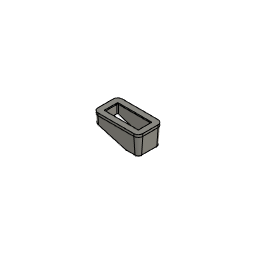
Power Switch Protector (Autodesk Fusion 360 design; units mm, degrees)
Autodesk Fusion 360 part; units mm, degrees
note: some values were not read from the file. Chosen so that the rebuilt part matches the saved one: a direction.
sketch "Sketch1" plane through (0, 0, 0) normal (0, 0, 1) x (-1, 0, 0)
  arc A0 (15.021, -6.6477) -> (15.275, -6.3937) centre (15.021, -6.3937) ccw
  line L0 (15.275, -6.3937) -> (15.275, 6.3937)
  arc A1 (15.275, 6.3937) -> (15.021, 6.6477) centre (15.021, 6.3937) ccw
  line L1 (15.021, 6.6477) -> (-15.021, 6.6477)
  arc A2 (-15.021, 6.6477) -> (-15.275, 6.3937) centre (-15.021, 6.3937) ccw
  line L2 (-15.275, 6.3937) -> (-15.275, -6.3937)
  arc A3 (-15.275, -6.3937) -> (-15.021, -6.6477) centre (-15.021, -6.3937) ccw
  line L3 (-15.021, -6.6477) -> (15.021, -6.6477)
  line L4 (17.675, -6.3937) -> (17.675, 6.3937)
  arc A4 (17.675, 6.3937) -> (15.021, 9.0477) centre (15.021, 6.3937) ccw
  line L5 (15.021, 9.0477) -> (-15.021, 9.0477)
  arc A5 (-15.021, 9.0477) -> (-17.675, 6.3937) centre (-15.021, 6.3937) ccw
  line L6 (-17.675, 6.3937) -> (-17.675, -6.3937)
  arc A6 (-17.675, -6.3937) -> (-15.021, -9.0477) centre (-15.021, -6.3937) ccw
  line L7 (-15.021, -9.0477) -> (15.021, -9.0477)
  arc A7 (15.021, -9.0477) -> (17.675, -6.3937) centre (15.021, -6.3937) ccw
  line L8 (15.675, -6.3937) -> (15.675, 6.3937)
  arc A8 (15.675, 6.3937) -> (15.021, 7.0477) centre (15.021, 6.3937) ccw
  line L9 (15.021, 7.0477) -> (-15.021, 7.0477)
  arc A9 (-15.021, 7.0477) -> (-15.675, 6.3937) centre (-15.021, 6.3937) ccw
  line L10 (-15.675, 6.3937) -> (-15.675, -6.3937)
  arc A10 (-15.675, -6.3937) -> (-15.021, -7.0477) centre (-15.021, -6.3937) ccw
  line L11 (-15.021, -7.0477) -> (15.021, -7.0477)
  arc A11 (15.021, -7.0477) -> (15.675, -6.3937) centre (15.021, -6.3937) ccw
  line L12 (15.021, 10.1477) -> (-15.021, 10.1477)
  arc A12 (-15.021, 10.1477) -> (-18.775, 6.3937) centre (-15.021, 6.3937) ccw
  line L13 (-18.775, 6.3937) -> (-18.775, -6.3937)
  arc A13 (-18.775, -6.3937) -> (-15.021, -10.1477) centre (-15.021, -6.3937) ccw
  line L14 (-15.021, -10.1477) -> (15.021, -10.1477)
  arc A14 (15.021, -10.1477) -> (18.775, -6.3937) centre (15.021, -6.3937) ccw
  line L15 (18.775, -6.3937) -> (18.775, 6.3937)
  arc A15 (18.775, 6.3937) -> (15.021, 10.1477) centre (15.021, 6.3937) ccw
  line L16 (-14.275, -5.6477) -> (14.275, -5.6477)
  line L17 (14.275, -5.6477) -> (14.275, 5.6477)
  line L18 (14.275, 5.6477) -> (-14.275, 5.6477)
  line L19 (-14.275, 5.6477) -> (-14.275, -5.6477)
  dimension "d2" = 2.4
  dimension "d5" = 0.4
  dimension "d8" = 3.5
  dimension "d16" = -1
extrude "Extrude1" add sketch "Sketch1" along normal blind 2 contours A0 L0 A1 L1 A2 L2 A3 L3 | L4 A4 L5 A5 L6 A6 L7 A7 | L8 A8 L9 A9 L10 A10 L11 A11
extrude "Extrude2" add sketch "Sketch1" against normal blind 15 contours L4 A4 L5 A5 L6 A6 L7 A7
extrude "Extrude3" add sketch "Sketch1" against normal blind 15 draft -4 contours L4 A4 L5 A5 L6 A6 L7 A7 | L12 A12 L13 A13 L14 A14 L15 A15
chamfer "Chamfer3" distance 8 distance2 25 1 edges at (-17.7261, 0, -15) measured on face at (-18.0757, 2.1312, -10)
fillet "Fillet1" radius 1 12 edges at (17.7261, 0, -15) (16.9338, 8.3064, -15) (11.1475, 9.0988, -15) (16.9338, -8.3064, -15) (11.1475, -9.0988, -15) (-3.8735, -9.3422, -11.5192) (-17.324, -8.6757, -7.3193) (-18.2841, 0, -7.0195) (-17.324, 8.6757, -7.3193) (-3.8735, 9.3422, -11.5192) (7.2739, -8.0732, -15) (7.2739, 8.0732, -15)
chamfer "Chamfer1" distance 0.6 angle 45 10 edges at (11.1475, -7.0477, -15) (15.4834, -6.8561, -15) (15.675, 0, -15) (15.4834, 6.8561, -15) (11.1475, 7.0477, -15) (-3.8735, -7.0477, -11.5192) (-3.8735, 7.0477, -11.5192) (-15.4834, 6.8561, -7.894) (-15.675, 0, -7.8342) (-15.4834, -6.8561, -7.894)
extrude "Extrude4" add sketch "Sketch1" along normal blind 2 contours L12 A12 L13 A13 L14 A14 L15 A15
fillet "Fillet2" radius 0.25 4 edges at (-14.275, 5.6477, 1) (-14.275, -5.6477, 1) (14.275, 5.6477, 1) (14.275, -5.6477, 1)
extrude "Extrude5" cut 1 faces at (4.675, -6.581, 0) along direction (0, 0, 1) blind 1
